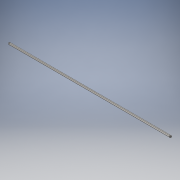
# Autodesk Inventor part: Main Axle
Saved by Autodesk Inventor 2019.4 (Build 234330000, 330)
## iProperties
Created: 2020-01-05
Part Number: Main Axle
Material: Steel, Mild
Document SubType Name: Modeling
Designer: admin
Density: 7.85 g/cm^3
Appearance: Semi-Polished
Author: admin
Autodesk Inventor part; units mm, degrees
ref_plane "YZ Plane" through (0, 0, 0) normal (1, 0, 0) x (0, 1, 0)
ref_plane "XZ Plane" through (0, 0, 0) normal (0, 1, 0) x (-1, 0, 0)
ref_plane "XY Plane" through (0, 0, 0) normal (0, 0, 1) x (1, 0, 0)
sketch "Sketch1" plane through (0, 0, 0) normal (0, 0, 1) x (1, 0, 0)
  line L0 (0, 0) -> (0, 4)
  line L1 (0, 4) -> (4, 4)
  line L2 (4, 4) -> (4, 5)
  line L3 (4, 5) -> (804, 5)
  line L4 (804, 5) -> (804, 4)
  line L5 (804, 4) -> (808, 4)
  line L6 (808, 4) -> (808, 0)
  line L7 (808, 0) -> (0, 0)
  dimension "d0" = 4
  dimension "d1" = 5
  dimension "d2" = 4
  dimension "d3" = 4
  dimension "d4" = 800
  constraints: 16 end point, 6 perpendicular, 2 point on line, 1 vertical
  measures "d0" distance of L0.start L0.end
  measures "d1" distance between parallel lines of L7 L3
  measures "d2" distance of L0.end L1.end
  measures "d3" distance of L4.end L5.end
  measures "d4" distance of L2.end L3.end
revolve "Revolution1" add sketch "Sketch1" angle 360 about axis through (808, 0, 0) along (-1, 0, 0)
body "Solid1"
